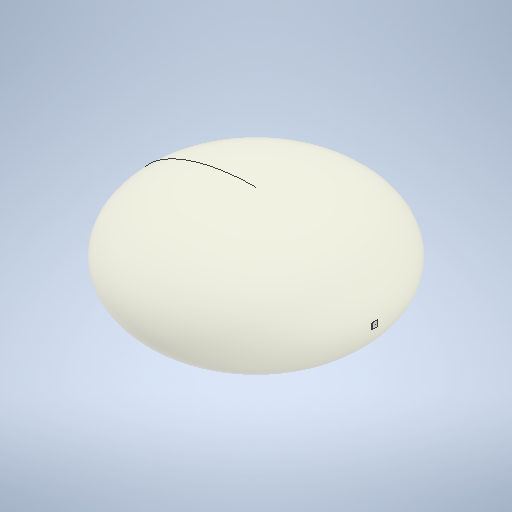
# Autodesk Inventor part: body
Saved by Autodesk Inventor 2025 (Build 290162010, 162A)
## iProperties
Created: 2025-08-07
Part Number: body
Material: 일반
Document SubType Name: Modeling
Designer: ytw32
Density: 1 g/cm^3
Appearance: 기본값
Author: ytw32
Autodesk Inventor part; units mm, degrees
ref_plane "XY Plane" through (0, 0, 0) normal (0, 0, 1) x (1, 0, 0)
sketch "스케치1" plane through (0, 0, 0) normal (0, 0, 1) x (1, 0, 0)
  spline S0 degree 5 poles (0, -500) (-87.9549, -499.9981) (-175.911, -495.1704) (-263.4968, -485.4852) (-384.3341, -464.9289) (-502.4081, -432.9377) (-535.292, -423.0038) (-591.5031, -404.1028) (-646.4777, -381.9053) (-669.3532, -371.9483) (-709.931, -352.8652) (-749.3336, -331.4776) (-766.5485, -321.5091) (-797.553, -302.2915) (-827.3287, -281.2305) (-840.5777, -271.2534) (-864.5807, -251.9247) (-887.2426, -231.0473) (-897.3858, -221.061) (-915.7565, -201.6202) (-932.6327, -180.8748) (-940.1627, -170.8774) (-953.7004, -151.3045) (-965.5664, -130.6802) (-970.7786, -120.6695) (-979.9524, -100.9336) (-987.2803, -80.4442) (-990.3483, -70.4203) (-995.4026, -50.4918) (-998.4798, -30.166) (-999.4933, -20.1333) (-1000.5067, 0) (-999.4933, 20.1333) (-998.4798, 30.166) (-995.4026, 50.4918) (-990.3483, 70.4203) (-987.2803, 80.4442) (-979.9524, 100.9336) (-970.7786, 120.6695) (-965.5664, 130.6802) (-953.7004, 151.3045) (-940.1627, 170.8774) (-932.6327, 180.8748) (-915.7565, 201.6202) (-897.3858, 221.061) (-887.2426, 231.0473) (-864.5807, 251.9247) (-840.5777, 271.2534) (-827.3287, 281.2305) (-797.553, 302.2915) (-766.5485, 321.5091) (-749.3336, 331.4776) (-709.931, 352.8652) (-669.3532, 371.9483) (-646.4777, 381.9053) (-591.5031, 404.1028) (-535.292, 423.0038) (-502.4081, 432.9377) (-384.3341, 464.9289) (-263.4968, 485.4852) (-175.911, 495.1704) (-87.9549, 499.9981) (0, 500) knots 0 0 0 0 0 0 0.181562 0.181562 0.181562 0.252435 0.252435 0.252435 0.303911 0.303911 0.303911 0.344954 0.344954 0.344954 0.37917 0.37917 0.37917 0.408531 0.408531 0.408531 0.434343 0.434343 0.434343 0.457612 0.457612 0.457612 0.479219 0.479219 0.479219 0.5 0.5 0.5 0.520781 0.520781 0.520781 0.542388 0.542388 0.542388 0.565657 0.565657 0.565657 0.591469 0.591469 0.591469 0.62083 0.62083 0.62083 0.655046 0.655046 0.655046 0.696089 0.696089 0.696089 0.747565 0.747565 0.747565 0.818438 0.818438 0.818438 1 1 1 1 1 1
  line L0 (0, 500) -> (0, -500)
  point P0 (0, 0)
  constraints: 2 end point, 1 vertical, 1 vertical alignment, 2 other
revolve "회전1" add sketch "스케치1" angle 360 about axis through (0, 500, 0) along (0, -1, 0)
ref_plane "작업 평면1" through (0, -500, 0) normal (0, 1, 0) x (-1, 0, 0)
sketch "스케치2" plane through (0, -500, 0) normal (0, 1, 0) x (-1, 0, 0)
  line L0 (50, -50) -> (-50, -50)
  line L1 (-50, -50) -> (-50, 50)
  line L2 (-50, 50) -> (50, 50)
  line L3 (50, 50) -> (50, -50)
  line L4 (50, -50) -> (-50, 50) construction
  line L5 (-50, -50) -> (50, 50) construction
  point P0 (0, 0)
  dimension "d7" = 100
  dimension "d8" = 100
  constraints: 12 end point, 2 midpoint, 2 parallel, 1 horizontal, 1 perpendicular
  measures "d7" distance of L1.end L2.end
  measures "d8" distance of L0.end L1.end
extrude "돌출1" add sketch "스케치2" along normal blind 10
ref_plane "작업 평면2" through (1000, 0, 0) normal (1, 0, 0) x (0, 1, 0)
sketch "스케치3" plane through (1000, 0, 0) normal (1, 0, 0) x (0, 1, 0)
  line L0 (25, 25) -> (-25, 25)
  line L1 (-25, 25) -> (-25, -25)
  line L2 (-25, -25) -> (25, -25)
  line L3 (25, -25) -> (25, 25)
  line L4 (25, 25) -> (-25, -25) construction
  line L5 (-25, 25) -> (25, -25) construction
  point P0 (0, 0)
  dimension "d12" = 50
  dimension "d13" = 50
  constraints: 12 end point, 2 midpoint, 2 parallel, 1 horizontal, 1 perpendicular
  measures "d12" distance of L2.end L1.end
  measures "d13" distance of L1.end L0.end
extrude "돌출2" add sketch "스케치3" against normal blind 10
pattern_circular "원형 패턴1" count 3 over 180 about axis through (0, -10, 0) along (0, 1, 0) of "돌출2"
equation "curve S0 of \"스케치1\": x = -sqrt(1000000 - 4 * t ^2); y = t; t from d3 to d4"
